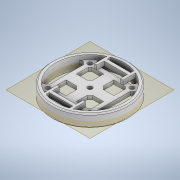
# Autodesk Inventor part: Electro_bat_up
Saved by Autodesk Inventor 2020 (Build 240168000, 168)
## iProperties
Created: 2020-09-03
Part Number: Electro_bat_up
Material: Generisch
Document SubType Name: Modeling
Designer: sp
Density: 1 g/cm^3
Appearance: Vorgabe
Author: sp
## iProperties of the stored document _3D-Druck.ipt
Created: 2020-09-03
Part Number: _3D-Druck
Material: Generisch
Document SubType Name: Modeling
Designer: sp
Density: 1 g/cm^3
Appearance: Vorgabe
Author: sp
Autodesk Inventor part; units mm, degrees
ref_plane "YZ Plane" through (0, 0, 0) normal (1, 0, 0) x (0, 1, 0)
ref_plane "XY Plane" through (0, 0, 0) normal (0, 0, 1) x (1, 0, 0)
sketch "Skizze1" plane through (0, 0, 0) normal (0, 1, 0) x (-1, 0, 0)
  circle A0 centre (0, 0) radius 30
  circle A1 centre (0, 0) radius 27
  dimension "d0" = 60
  dimension "d1" = 54
  constraints: 2 centre point, 2 coincident
  measures "d0" diameter of A0
  measures "d1" diameter of A1
extrude "Extrusion1" add sketch "Skizze1" along normal mid plane 10
ref_plane "Arbeitsebene1" through (0, 0, 0) normal (0, 1, 0) x (-1, 0, 0)
chamfer "Fase1" distance 1 angle 45 2 edges at (30, 5, 0) (30, -5, 0)
sketch "Skizze2" plane through (0, 0, 0) normal (0, 1, 0) x (-1, 0, 0)
  line L0 (0, 42.2301) -> (0, -36.7007) construction
  line L1 (32.6355, 0) -> (-32.6355, 0) construction
  line L2 (16.5, 34.419) -> (16.5, -40.3324) construction
  line L3 (-16.5, 35.4304) -> (-16.5, -34.8157) construction
  line L4 (23.5881, 16.5) -> (-32.0387, 16.5) construction
  line L5 (23.5881, -16.5) -> (-39.8541, -16.5) construction
  circle A0 centre (16.5, -16.5) radius 1.75
  circle A1 centre (16.5, 16.5) radius 1.75
  circle A2 centre (-16.5, 16.5) radius 1.75
  circle A3 centre (-16.5, -16.5) radius 1.75
  circle A4 centre (-16.5, 16.5) radius 3.6749
  circle A5 centre (-16.5, -16.5) radius 3.7161
  circle A6 centre (16.5, -16.5) radius 3.7
  circle A7 centre (16.5, 16.5) radius 3.6747
  point P0 (0, 0)
  dimension "d8" = 33
  dimension "d9" = 33
  dimension "d10" = 3.5
  dimension "d11" = 3.5
  dimension "d12" = 3.5
  dimension "d13" = 3.5
  constraints: 12 end point, 9 point on line, 8 centre point, 4 coincident, 3 horizontal, 3 vertical, 1 midpoint, 2 other
  measures "d8" distance between parallel lines of L3 L2
  measures "d9" distance between parallel lines of L4 L5
  measures "d10" diameter of A0
  measures "d11" diameter of A1
  measures "d12" diameter of A2
  measures "d13" diameter of A3
extrude "Extrusion2" add sketch "Skizze2" along normal mid plane 3
fillet "Rundung1" radius 2 16 edges at (-18.7043, 0.75, -19.4718) (-18.7043, -0.75, -19.4718) (-19.4718, 0.75, -18.7043) (-19.4718, -0.75, -18.7043) (-18.8927, 0.75, 19.289) (-18.8927, -0.75, 19.289) (-19.289, 0.75, 18.8927) (-19.289, -0.75, 18.8927) (18.8904, 0.75, 19.2913) (18.8904, -0.75, 19.2913) (19.2913, 0.75, 18.8904) (19.2913, -0.75, 18.8904) (19.551, 0.75, -18.6215) (19.551, -0.75, -18.6215) (18.6215, 0.75, -19.551) (18.6215, -0.75, -19.551)
sketch "Skizze3" plane through (0, 0, 0) normal (0, 1, 0) x (-1, 0, 0)
  circle A0 centre (-16.5, -16.5) radius 1.75 projected
  line L0 (16.5712, -18.25) -> (-16.5, -18.25)
  line L1 (-16.5, -18.25) -> (-16.5, -14.75)
  line L2 (-16.5, -14.75) -> (16.5712, -14.75)
  line L3 (16.5712, -14.75) -> (16.5712, -18.25)
  circle A1 centre (-16.5, 16.5) radius 1.75 projected
  line L4 (-18.25, 16.5) -> (-14.75, 16.5)
  line L5 (-14.75, 16.5) -> (-14.75, -16.5)
  line L6 (-14.75, -16.5) -> (-18.25, -16.5)
  line L7 (-18.25, -16.5) -> (-18.25, 16.5)
  circle A2 centre (16.5, 16.5) radius 1.75 projected
  line L8 (16.5, 14.75) -> (-16.8045, 14.75)
  line L9 (-16.8045, 14.75) -> (-16.8045, 18.2233)
  line L10 (-16.8045, 18.2233) -> (16.5, 18.2233)
  line L11 (16.5, 18.2233) -> (16.5, 14.75)
  circle A3 centre (-16.5, -16.5) radius 1.75 projected
  circle A4 centre (16.5, -16.5) radius 1.75 projected
  line L12 (18.25, -16.5) -> (14.75, -16.5)
  line L13 (14.75, -16.5) -> (14.75, 16.5)
  line L14 (14.75, 16.5) -> (18.25, 16.5)
  line L15 (18.25, 16.5) -> (18.25, -16.5)
  point P0 (0, 0)
  point P1 (14.75, -14.75)
  point P2 (-14.75, -14.75)
  point P3 (16.5, -18.25)
  point P4 (14.75, 14.75)
  point P5 (16.1955, 18.2233)
  point P6 (-16.1955, 18.2233)
  point P7 (-14.75, 14.75)
  point P8 (16.5712, -14.7514)
  point P9 (-16.8045, 14.7767)
  constraints: 32 end point, 8 parallel, 7 point on circle, 4 horizontal, 4 perpendicular, 2 other
extrude "Extrusion3" add sketch "Skizze3" against normal mid plane 3 contours L5 L2 L13 A4 L0 A0 | A0 L7 A1 L9 L8 L5 L2 | L13 L8 A2 L15 A4 L2 | L5 A1 L10 A2 L13 L8
sketch "Skizze4" plane through (0, 1.5, 0) normal (0, 1, 0) x (1, 0, 0)
  line L0 (0, 40.2437) -> (0, -26.2031) construction
  line L1 (9.25, 25.7) -> (11.25, 25.7)
  line L2 (11.25, 25.7) -> (11.25, 14.7)
  line L3 (11.25, 14.7) -> (9.25, 14.7)
  line L4 (9.25, 14.7) -> (9.25, 25.7)
  line L5 (-11.25, 25.7) -> (-9.25, 25.7)
  line L6 (-9.25, 25.7) -> (-9.25, 14.7)
  line L7 (-9.25, 14.7) -> (-11.25, 14.7)
  line L8 (-11.25, 14.7) -> (-11.25, 25.7)
  point P0 (0, 0)
  dimension "d19" = 2
  dimension "d20" = 2
  dimension "d21" = 18.5
  dimension "d22" = 14.7
  dimension "d23" = 11
  dimension "d24" = 11
  dimension "d25" = 14.7
  constraints: 18 end point, 4 parallel, 2 horizontal, 2 perpendicular, 1 point on line, 1 vertical, 1 other
  measures "d19" distance of L6.end L7.end
  measures "d20" distance of L2.end L3.end
  measures "d21" distance between parallel lines of L6 L4
  measures "d22" distance from line of point (0, 0) L3
  measures "d23" distance of L1.end L2.end
  measures "d24" distance of L5.end L6.end
  measures "d25" distance from line of point (0, 0) L7
extrude "Extrusion4" add sketch "Skizze4" along normal blind 3.5
mirror "Spiegeln1" about plane through (0, 0, 0) normal (0, 0, 1) of "Extrusion4"
sketch "Skizze5" plane through (0, 5, 0) normal (0, 1, 0) x (1, 0, 0)
  line L0 (-46.6461, 0) -> (88.9964, 0) construction
  line L1 (-9.25, 18.25) -> (-9.25, 25.3661) projected
  line L2 (9.25, 25.3661) -> (9.25, 18.25) projected
  line L3 (-9.25, 22.75) -> (9.25, 22.75)
  line L4 (9.25, 22.75) -> (9.25, 20.25)
  line L5 (9.25, 20.25) -> (-9.25, 20.25)
  line L6 (-9.25, 20.25) -> (-9.25, 22.75)
  line L7 (-9.25, -14.7) -> (-9.25, -25.3661) projected
  line L8 (-9.25, -22.75) -> (9.25, -22.75)
  line L9 (9.25, -22.75) -> (9.25, -20.25)
  line L10 (9.25, -20.25) -> (-9.25, -20.25)
  line L11 (-9.25, -20.25) -> (-9.25, -22.75)
  point P0 (0, 0)
  point P1 (-9.25, 20.25)
  dimension "d28" = 2.5
  dimension "d29" = 40.5
  dimension "d30" = 2.5
  constraints: 18 end point, 4 parallel, 4 point on line, 3 horizontal, 2 perpendicular, 1 other
  measures "d28" distance between parallel lines of L8 L10
  measures "d29" distance between parallel lines of L10 L5
  measures "d30" distance between parallel lines of L5 L3
extrude "Extrusion5" add sketch "Skizze5" against normal blind 3.5
sketch "Skizze7" plane through (0, -1.5, 0) normal (0, -1, 0) x (1, 0, 0)
  circle A0 centre (0, 0) radius 1.75
  circle A1 centre (0, 0) radius 7.5
  line L0 (-9.25, -14.75) -> (9.25, -14.75) projected
  line L1 (4, -14.75) -> (-4, -14.75)
  line L2 (-4, -14.75) -> (-4, -6.3443)
  line L3 (-4, -6.3443) -> (4, -6.3443)
  line L4 (4, -6.3443) -> (4, -14.75)
  point P0 (-4, -14.75)
  dimension "d36" = 15
  dimension "d35" = 3.5
  dimension "d37" = 8
  dimension "d38" = 4
  constraints: 8 end point, 2 coincident, 2 parallel, 1 centre point, 1 horizontal, 1 perpendicular, 1 point on line, 3 other
  measures "d35" diameter of A0
  measures "d37" distance between parallel lines of L2 L4
  measures "d38" distance from line of point (0, 0) L2
extrude "Extrusion7" add sketch "Skizze7" against normal blind 3
pattern_circular "Runde Anordnung1" count 4 over 360 about axis through (0, -10, 0) along (0, 1, 0) of "Extrusion7"
